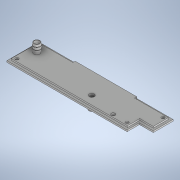
# Autodesk Inventor part: Klapa
Saved by Autodesk Inventor 2022 (Build 260153000, 153)
## iProperties
Created: 2022-08-24
Part Number: Klapa
Material: Ogólny
Document SubType Name: Modeling
Designer: kosak
Density: 1 g/cm^3
Appearance: Domyślna
Author: kosak
## iProperties of the stored document Klapa_Drukowanie 3D.ipt
Created: 2022-10-04
Part Number: Klapa_Drukowanie 3D
Material: Ogólny
Document SubType Name: Modeling
Designer: kosak
Density: 1 g/cm^3
Appearance: Domyślna
Author: kosak
Autodesk Inventor part; units mm, degrees
sketch "Szkic1" plane through (0, 0, 0) normal (0, 1, 0) x (-1, 0, 0)
  line L0 (0, 0) -> (-174, 0)
  line L1 (-174, 0) -> (-174, -41.646)
  line L2 (-174, -41.646) -> (0, -41.646)
  line L3 (0, -41.646) -> (0, 0)
  dimension "d0" = 174
  dimension "d1" = 41.646
  constraints: 8 end point, 2 parallel, 1 horizontal, 1 perpendicular
  measures "d0" distance of L2.end L1.end
  measures "d1" distance of L1.end L0.end
extrude "Wyciągnięcie proste1" add sketch "Szkic1" along normal blind 2
sketch "Szkic2" plane through (0, 2, 0) normal (0, 1, 0) x (1, 0, 0)
  line L0 (174, 41.646) -> (0, 41.646) projected
  line L1 (174, 0) -> (174, 41.646) projected
  line L2 (174, 41.646) -> (0, 41.646) projected
  line L3 (0, 41.646) -> (0, 0) projected
  line L4 (0, 0) -> (174, 0) projected
  line L5 (171, 23) -> (171, 38.646)
  line L6 (2.5, 38.646) -> (2.5, 3)
  line L7 (2.5, 3) -> (153.5, 3)
  line L8 (2.5, 41.646) -> (2.5, 38.646)
  line L9 (127, 41.646) -> (47, 41.646)
  line L10 (153.5, 19) -> (171, 19)
  line L11 (171, 19) -> (171, 23)
  line L12 (153.5, 19) -> (153.5, 3)
  line L13 (127, 38.646) -> (127, 41.646)
  line L14 (2.5, 38.646) -> (47, 38.646)
  line L15 (127, 38.646) -> (171, 38.646)
  line L16 (47, 38.646) -> (47, 41.646)
  dimension "d4" = 3
  dimension "d122" = 17.5
  dimension "d123" = 16
  dimension "d150" = 3
  dimension "d151" = 44.5
  constraints: 24 end point, 5 perpendicular, 3 vertical, 2 horizontal, 1 collinear, 1 point on line
  measures "d4" distance between parallel lines of L4 L7
  measures "d122" distance of L10.start L10.end
  measures "d123" distance of L10.start L7.end
  measures "d150" distance of L13.start L9.start
  measures "d151" distance of L6.start L14.end
extrude "Wyciągnięcie proste2" add sketch "Szkic2" along normal blind 2 contours L13 L15 L5 L11 L10 L12 L7 L6 L14 L16 L0
sketch "Szkic21" plane through (0, 0, 0) normal (0, -1, 0) x (1, 0, 0)
  line L0 (0, -41.646) -> (0, 0) projected
  line L1 (0, -41.646) -> (0, 0) projected
  line L2 (0, -26.646) -> (12, -26.646)
  line L3 (174, -41.646) -> (0, -41.646) projected
  line L4 (12, -41.646) -> (12, -26.646)
  circle A0 centre (12, -26.646) radius 3.9
  dimension "d90" = 12
  dimension "d91" = 15
  dimension "d92" = 7.8
  constraints: 4 end point, 2 point on line, 1 centre point, 1 coincident, 1 perpendicular, 1 vertical
  measures "d90" distance of L2.end L2.start
  measures "d91" distance of L4.start L2.end
  measures "d92" diameter of A0
extrude "Wyciągnięcie proste20" add sketch "Szkic21" along normal blind 5 contours A0 L4 L2 | L2 L4 A0
sketch "Szkic22" plane through (12, -5, -26.646) normal (0, -1, 0) x (1, 0, 0)
  circle A0 centre (0, 0) radius 3.9
  circle A1 centre (0.19341, 0) radius 4.4
  point P0 (-12, 26.646)
  dimension "d95" = 8.8
  constraints: 1 centre point
  measures "d95" diameter of A1
extrude "Wyciągnięcie proste21" add sketch "Szkic22" along normal blind 0.5 contours A0 | A1
ref_plane "Płaszczyzna konstrukcyjna1" through (12.19341, -5.5, -26.646) normal (0, -1, 0) x (1, 0, 0)
sketch "Szkic23" plane through (12.19341, -5.5, -26.646) normal (0, -1, 0) x (1, 0, 0)
  circle A0 centre (0, 0) radius 4.4 projected
  circle A1 centre (0, 0) radius 4.4
  point P0 (-12.19341, 26.646)
  constraints: 1 centre point, 1 coincident
extrude "Wyciągnięcie proste22" add sketch "Szkic23" along normal blind 2.5 draft -11.31
sketch "Szkic24" plane through (12.19341, -8, -26.646) normal (0, -1, 0) x (1, 0, 0)
  circle A0 centre (0, 0) radius 3.899997
  circle A1 centre (0, 0) radius 3.899997
  point P0 (-12.19341, 26.646)
  constraints: 1 centre point, 1 coincident, 1 concentric
extrude "Wyciągnięcie proste23" add sketch "Szkic24" along normal blind 0.5
sketch "Szkic25" plane through (12.19341, -8.5, -26.646) normal (0, -1, 0) x (1, 0, 0)
  circle A0 centre (0, 0) radius 4.4 projected
  circle A1 centre (0, 0) radius 4.4
  point P0 (-12.19341, 26.646)
  constraints: 1 centre point, 1 coincident, 1 concentric
extrude "Wyciągnięcie proste24" add sketch "Szkic25" along normal blind 0.5
ref_plane "Płaszczyzna konstrukcyjna2" through (12.19341, -9, -26.646) normal (0, -1, 0) x (1, 0, 0)
sketch "Szkic26" plane through (12.19341, -9, -26.646) normal (0, -1, 0) x (1, 0, 0)
  circle A0 centre (0, 0) radius 4.4 projected
  circle A1 centre (0, 0) radius 4.4
  point P0 (-12.19341, 26.646)
  constraints: 1 centre point, 1 coincident, 1 concentric
extrude "Wyciągnięcie proste25" add sketch "Szkic26" along normal blind 2.5 draft -11.31
sketch "Szkic27" plane through (12.19341, -11.5, -26.646) normal (0, -1, 0) x (1, 0, 0)
  circle A0 centre (0, 0) radius 3.899997
  circle A1 centre (0, 0) radius 3.25
  point P0 (-12.19341, 26.646)
  dimension "d108" = 6.5
  constraints: 1 centre point, 1 coincident
  measures "d108" diameter of A1
extrude "Wyciągnięcie proste26" cut sketch "Szkic27" against normal blind 32 contours A1
mirror "Odbij1" about plane through (87, 2, -20.823) normal (0, 1, 0) of "Wyciągnięcie proste20", "Wyciągnięcie proste21", "Wyciągnięcie proste22", "Wyciągnięcie proste24", "Wyciągnięcie proste25", "Wyciągnięcie proste26", "Wyciągnięcie proste23"
sketch "Szkic28" plane through (0, 0, 0) normal (0, -1, 0) x (1, 0, 0)
  line L0 (174, 0) -> (174, -41.646) projected
  line L1 (174, 0) -> (156, 0)
  line L2 (156, 0) -> (156, -16)
  line L3 (156, -16) -> (174, -16)
  line L4 (174, -16) -> (174, 0)
  point P0 (0, 0)
  dimension "d111" = 18
  dimension "d112" = 16
  constraints: 8 end point, 2 parallel, 1 horizontal, 1 perpendicular
  measures "d111" distance of L3.end L2.end
  measures "d112" distance of L2.end L1.end
extrude "Wyciągnięcie proste27" cut sketch "Szkic28" against normal blind 4
sketch "Szkic29" plane through (0, 0, 0) normal (0, -1, 0) x (1, 0, 0)
  line L0 (0, 0) -> (156, 0) projected
  line L1 (0, 0) -> (96.2, 0)
  line L2 (96.2, 0) -> (96.2, -14)
  circle A0 centre (96.2, -14) radius 3.9
  dimension "d124" = 96.2
  dimension "d125" = 14
  dimension "d126" = 7.8
  constraints: 4 end point, 1 centre point, 1 coincident, 1 point on line, 1 vertical
  measures "d124" distance of L0.start L1.end
  measures "d125" distance of L1.end L2.end
  measures "d126" diameter of A0
extrude "Wyciągnięcie proste28" add sketch "Szkic29" along normal blind 5
sketch "Szkic30" plane through (96.2, -5, -14) normal (0, -1, 0) x (1, 0, 0)
  circle A0 centre (0, 0) radius 3.9 projected
  circle A1 centre (0, 0) radius 4.4
  point P0 (-96.2, 14)
  dimension "d129" = 8.8
  constraints: 1 centre point, 1 coincident
  measures "d129" diameter of A1
extrude "Wyciągnięcie proste29" add sketch "Szkic30" along normal blind 0.5 contours A0 | A1
ref_plane "Płaszczyzna konstrukcyjna3" through (96.2, -5.5, -14) normal (0, -1, 0) x (1, 0, 0)
sketch "Szkic31" plane through (96.2, -5.5, -14) normal (0, -1, 0) x (1, 0, 0)
  circle A0 centre (0, 0) radius 4.4 projected
  circle A1 centre (0, 0) radius 4.4
  point P0 (-96.2, 14)
  constraints: 1 centre point, 1 coincident
extrude "Wyciągnięcie proste30" add sketch "Szkic31" along normal blind 2.5 draft -11.31
sketch "Szkic32" plane through (96.2, -8, -14) normal (0, -1, 0) x (1, 0, 0)
  circle A0 centre (0, 0) radius 3.899997
  point P0 (-96.2, 14)
  constraints: 1 centre point
extrude "Wyciągnięcie proste31" add sketch "Szkic32" along normal blind 0.5
sketch "Szkic33" plane through (96.2, -8.5, -14) normal (0, -1, 0) x (1, 0, 0)
  circle A0 centre (0, 0) radius 4.4 projected
  circle A1 centre (0, 0) radius 4.4
  point P0 (-96.2, 14)
  constraints: 1 centre point, 1 coincident
extrude "Wyciągnięcie proste32" add sketch "Szkic33" along normal blind 0.5
ref_plane "Płaszczyzna konstrukcyjna4" through (96.2, -9, -14) normal (0, -1, 0) x (1, 0, 0)
sketch "Szkic34" plane through (96.2, -9, -14) normal (0, -1, 0) x (1, 0, 0)
  circle A0 centre (0, 0) radius 3.9 projected
  circle A1 centre (0, 0) radius 4.4
  point P0 (-96.2, 14)
  constraints: 1 centre point, 1 coincident
sketch "Szkic34 outline for Wyciągnięcie proste33" plane through (96.2, -9, -14) normal (0, -1, 0) x (1, 0, 0)
  circle A0 centre (0, 0) radius 4.4
extrude "Wyciągnięcie proste33" add sketch "Szkic34 outline for Wyciągnięcie proste33" along normal blind 2.5 draft -11.31
sketch "Szkic35" plane through (96.2, -11.5, -14) normal (0, -1, 0) x (1, 0, 0)
  circle A0 centre (0, 0) radius 3.25
  point P0 (-96.2, 14)
  dimension "d142" = 6.5
  constraints: 1 centre point
  measures "d142" diameter of A0
extrude "Wyciągnięcie proste34" cut sketch "Szkic35" against normal blind 16
sketch "Szkic37" plane through (0, 0, 0) normal (0, -1, 0) x (1, 0, 0)
  line L0 (0, 0) -> (156, 0)
  line L1 (2.5, -3) -> (153.5, -3)
  line L2 (0, -6.5) -> (6.5, -6.5)
  line L3 (6.5, 0) -> (6.5, -6.5)
  line L4 (0, -41.646) -> (0, 0)
  circle A0 centre (6.5, -6.5) radius 3
  line L5 (0, -20.823) -> (4.213625, -20.823)
  circle A1 centre (6.5, -35.146) radius 3
  line L6 (174, -41.646) -> (0, -41.646)
  line L7 (87, -41.646) -> (87, -34.846)
  circle A2 centre (167.5, -35.146) radius 3
  line L8 (2.5, -3) -> (78, -3)
  line L9 (78, -3) -> (78, -5.430935)
  circle A3 centre (149.5, -6.5) radius 3
  dimension "d156" = 6.5
  dimension "d160" = 6.5
  dimension "d161" = 6
  constraints: 12 end point, 4 centre point, 3 midpoint, 3 symmetric about line, 2 horizontal, 2 point on line, 2 vertical, 1 coincident, 1 perpendicular, 3 other
  measures "d156" distance of L2.end L2.start
  measures "d160" distance of L3.start L2.end
  measures "d161" diameter of A0
extrude "Wyciągnięcie proste37" cut sketch "Szkic37" against normal blind 2.8 contours A0 L3 L2 | L2 L3 A0 | A1 | A2 | A3
sketch "Szkic38" plane through (6.5, 2.8, -6.5) normal (0, -1, 0) x (1, 0, 0)
  circle A0 centre (0, 0) radius 2
  line L0 (-6.5, -35.146) -> (-6.5, 6.5) projected
  line L1 (-6.5, -14.323) -> (-2.3, -14.323)
  circle A1 centre (0, -28.646) radius 2
  line L2 (167.5, -35.146) -> (-6.5, -35.146) projected
  line L3 (80.5, -35.146) -> (80.5, -30.046)
  circle A2 centre (161, -28.646) radius 2
  line L4 (-4, 3.5) -> (147, 3.5) projected
  line L5 (-4, 3.5) -> (71.5, 3.5)
  line L6 (71.5, 3.5) -> (71.5, -1.9)
  circle A3 centre (143, 0) radius 2
  dimension "d164" = 4
  constraints: 8 end point, 4 centre point, 3 midpoint, 3 symmetric about line, 2 vertical, 1 horizontal, 3 other
  measures "d164" diameter of A0
extrude "Wyciągnięcie proste38" cut sketch "Szkic38" against normal blind 3
sketch "Szkic39" plane through (0, 0, 0) normal (0, -1, 0) x (1, 0, 0)
  circle A0 centre (149.5, -6.5) radius 3 projected
  line L0 (146.5, -6.5) -> (131.5, -6.5)
  circle A1 centre (131.5, -6.5) radius 2.5
  point P0 (0, 0)
  dimension "d167" = 15
  dimension "d168" = 5
  constraints: 2 end point, 1 centre point, 1 coincident, 1 horizontal, 1 horizontal alignment, 1 other
  measures "d167" distance of L0.start L0.end
  measures "d168" diameter of A1
extrude "Wyciągnięcie proste39" cut sketch "Szkic39" against normal blind 10 contours A1
